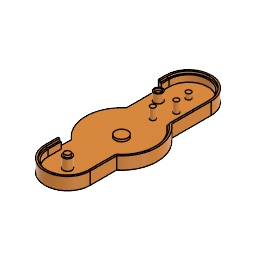
LowerHousing (Autodesk Fusion 360 design; units mm, degrees)
part number: 2026-05-31-18-17-23-774
Autodesk Fusion 360 part; units mm, degrees
sketch "Sketch1" plane through (0, 0, 0) normal (0, 0, 1) x (1, 0, 0)
  circle A0 centre (0, 0) radius 2.9
  circle A1 centre (0, 0) radius 12 construction
  line L0 (0, -25) -> (0, 0) construction
  circle A2 centre (0, 14.5) radius 6 construction
  line L1 (0, 0) -> (0, 12) construction
  circle A3 centre (0, 14.5) radius 2.5 construction
  circle A4 centre (0, 31) radius 4.5 construction
  circle A5 centre (2.9141, 22.4848) radius 2.5 construction
  circle A6 centre (2.9141, 22.4848) radius 4.5 construction
  line L2 (0, 14.5) -> (0, 12) construction
  line L3 (-9, -25) -> (-9, -12)
  line L4 (-9, 12) -> (-9, 31)
  line L5 (9, -25) -> (9, -12)
  line L6 (9, 12) -> (9, 31)
  arc A7 (-9, -25) -> (9, -25) centre (0, -25) ccw
  arc A8 (-9, 12) -> (-9, -12) centre (0, 0) ccw
  arc A9 (9, -12) -> (9, 12) centre (0, 0) ccw
  arc A10 (9, 31) -> (-9, 31) centre (0, 31) ccw
  circle A11 centre (0, 14.5) radius 1.15
  circle A12 centre (2.9141, 22.4848) radius 1.15
  circle A13 centre (0, 31) radius 1.15
  line L7 (-6, 23) -> (-9, 23) construction
  circle A14 centre (-6, 23) radius 1.95
  arc A15 (10.5, 31) -> (-10.5, 31) centre (0, 31) ccw
  line L8 (-10.5, 12.7279) -> (-10.5, 31)
  arc A16 (-10.5, 12.7279) -> (-10.5, -12.7279) centre (0, 0) ccw
  line L9 (-10.5, -25) -> (-10.5, -12.7279)
  arc A17 (-10.5, -25) -> (10.5, -25) centre (0, -25) ccw
  line L10 (10.5, -25) -> (10.5, -12.7279)
  arc A18 (10.5, -12.7279) -> (10.5, 12.7279) centre (0, 0) ccw
  line L11 (10.5, 12.7279) -> (10.5, 31)
  line L12 (-10.5, -18.864) -> (-9, -18.864)
  line L13 (-9, 21.5) -> (-10.5, 21.5) construction
  line L14 (-9, 27.5) -> (-10.5, 27.5)
  line L15 (-9.7, -25) -> (-9.7, -18.864)
  arc A19 (-9.7, -25) -> (9.7, -25) centre (0, -25) ccw
  line L16 (9.7, -25) -> (9.7, -12.345)
  arc A20 (9.7, -12.345) -> (9.7, 12.345) centre (0, 0) ccw
  line L17 (9.7, 12.345) -> (9.7, 31)
  arc A21 (9.7, 31) -> (-9.7, 31) centre (0, 31) ccw
  line L18 (-9.7, 27.5) -> (-9.7, 31)
  circle A22 centre (0, -25) radius 2
  circle A23 centre (0, -25) radius 1.325
  circle A24 centre (-6, 23) radius 1.425
  dimension "d1" = 56
  dimension "d2" = 30
  dimension "d4" = 18
  dimension "d5" = 18
  dimension "d6" = 5.8
  dimension "d11" = 24
  dimension "d12" = 25
  dimension "d13" = 12
  dimension "d14" = 5
  dimension "d15" = 9
  dimension "d16" = 5
  dimension "d18" = 9
  dimension "d19" = 15
  dimension "d20" = 2.3
  dimension "d21" = 2.3
  dimension "d22" = 2.3
  dimension "d26" = 3
  dimension "d27" = 8
  dimension "d28" = 3.9
  dimension "d31" = 1.5
  dimension "d32" = 6
  dimension "d38" = 15.7
  dimension "d39" = 9.7
  dimension "d40" = 4
  dimension "d41" = 2.65
  dimension "d42" = 2.85
  dimension "d58" = 9.7
  constraint coincident A0.centre A1.centre
  constraint tangent L4 A10
  constraint tangent L6 A10
  constraint concentric A1 A8
  constraint parallel L3 L5
  constraint vertical L3
  constraint coincident L0.start A7.centre
  constraint parallel L0 L5
  constraint parallel L0 L1
  constraint concentric A2 A3
  constraint concentric A4 A10
  constraint tangent A2 A5
  constraint concentric A5 A6
  constraint tangent A4 A6
  constraint coincident A2.centre A3.centre
  constraint coincident A3 L1.end
  constraint vertical L2
  constraint coincident A1 L1.end
  constraint collinear L3 L4
  constraint collinear L5 L6
  constraint concentric A8 A9
  constraint concentric A2 A11
  constraint concentric A5 A12
  constraint concentric A4 A13
  constraint horizontal L7
  constraint coincident L7.start A14.centre
  constraint coincident L4 L7.end
  constraint midpoint L9 L12.start
  constraint coincident L3 L12.end
  constraint perpendicular L3 L12
  constraint midpoint L4 L13.start
  constraint coincident L8 L13.end
  constraint perpendicular L8 L13
  constraint coincident L4 L14.start
  constraint coincident L8 L14.end
  constraint concentric A7 A19
  constraint concentric A9 A20
  constraint concentric A10 A21
  constraint coincident L12 L15.end
  constraint coincident L14 L18.start
  constraint concentric A7 A22
  constraint concentric A22 A23
  constraint concentric A14 A24
  measures "d1" distance of L0.start A4.centre
  measures "d2" diameter of A8
  measures "d4" diameter of A10
  measures "d5" diameter of A7
  measures "d6" diameter of A0
  measures "d11" diameter of A1
  measures "d12" distance of L0.start A0.centre
  measures "d13" diameter of A2
  measures "d14" diameter of A3
  measures "d15" diameter of A4
  measures "d16" diameter of A5
  measures "d18" diameter of A6
  measures "d19" radius of A9
  measures "d20" diameter of A11
  measures "d21" diameter of A12
  measures "d22" diameter of A13
  measures "d26" distance of L7.start L7.end
  measures "d27" distance of A4.centre L7
  measures "d28" diameter of A14
  measures "d38" radius of A20
  measures "d39" radius of A19
  measures "d40" diameter of A22
  measures "d41" diameter of A23
  measures "d42" diameter of A24
  measures "d58" radius of A21
extrude "Extrude1" add sketch "Sketch1" along normal blind 2 contours L3 L4 L5 L6 A7 A8 A9 A10 | A11 | A12 | A13 | A14 | A22 | A23 | A24 makes body 1
extrude "Extrude2" add sketch "Sketch1" along normal blind 3 contours A0 bodies 1
extrude "Extrude3" add sketch "Sketch1" along normal blind 7 contours A11 | A12 | A13 bodies 1
extrude "Extrude4" add sketch "Sketch1" along normal blind 6 contours A14 | A24 bodies 1
extrude "Extrude5" add sketch "Sketch1" along normal blind 6 separate body contours A15 L8 L9 A17 L10 A18 L11 L12 L14 L15 A19 L16 A20 L17 A21 L18 makes body 2
extrude "Extrude6" add sketch "Sketch1" along normal blind 2 contours L3 L4 A8 L8 A16 L9 L12 L14 bodies 1
extrude "Extrude7" add sketch "Sketch1" along normal blind 5 contours L3 L4 L5 L6 A7 A9 A10 L12 L14 L15 A19 L16 A20 L17 A21 L18 bodies 1 2
extrude "Extrude8" cut 1 faces at (-0.5421, 30.7672, 7) along direction (0, 0, -1) blind 2.5 on bodies 1 bodies 1
extrude "Extrude9" cut sketch "Sketch1" along normal blind 3 from surface at 5 contours A24 bodies 1
extrude "Extrude10" add sketch "Sketch1" along normal blind 7 contours A22 | A23 bodies 1
extrude "Extrude11" add sketch "Sketch1" along normal blind 8 contours A23 bodies 1
fillet "Fillet1" radius 0.25 8 edges at (-10.5, -18.864, 0) (0, -35.5, 0) (10.5, -18.864, 0) (16.5, 0, 0) (10.5, 21.864, 0) (0, 41.5, 0) (-10.5, 21.864, 0) (-16.5, 0, 0) on bodies 1
equation "d5 = d4"
